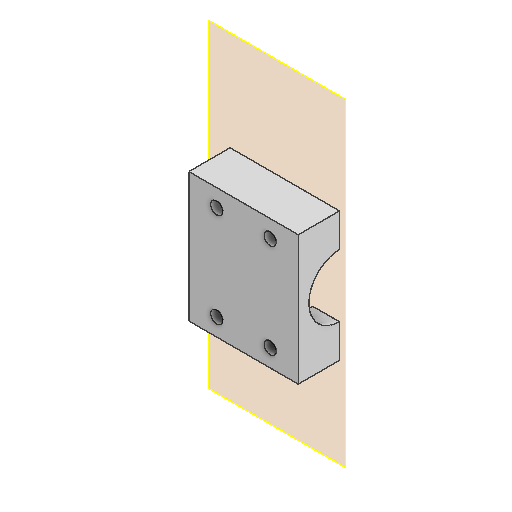
# Autodesk Inventor part: Cuvette Holder Transmit Holddown
Saved by Autodesk Inventor 2025.1 (Build 291241020, 241B)
## iProperties
Created: 2024-09-23
Part Number: Cuvette Holder Transmit Holddown
Material: Generic
Document SubType Name: Modeling
Designer: wayneslade
Density: 1 g/cm^3
Appearance: Default
Author: wayneslade
Autodesk Inventor part; units mm, degrees
ref_plane "YZ Plane" through (0, 0, 0) normal (1, 0, 0) x (0, 1, 0)
ref_plane "XZ Plane" through (0, 0, 0) normal (0, 1, 0) x (-1, 0, 0)
ref_plane "Work Plane1" through (0, 0, 0) normal (0, 0, 1) x (1, 0, 0)
sketch "Sketch1" plane through (0, 0, 0) normal (0, 0, 1) x (1, 0, 0)
  circle A0 centre (13.9438, -25.4) radius 3.3782 construction
  line L0 (31.1796, -40) -> (-0.106, -40) construction
  line L1 (31.1796, -40) -> (31.1796, -8.95) construction
  line L2 (31.1796, -8.95) -> (23.5548, -8.95) construction
  line L3 (23.5548, -8.95) -> (23.5548, -10.525) construction
  line L4 (23.5548, -10.525) -> (12.648, -10.525) construction
  line L5 (12.648, -10.525) -> (12.648, -8.95) construction
  line L6 (12.648, -8.95) -> (-0.106, -8.95) construction
  line L7 (-0.106, -8.95) -> (-0.106, -40) construction
  circle A1 centre (13.9438, 25.4) radius 3.3782 construction
  line L8 (-0.106, 8.95) -> (12.648, 8.95) construction
  line L9 (12.648, 8.95) -> (12.648, 10.525) construction
  line L10 (12.648, 10.525) -> (23.5548, 10.525) construction
  line L11 (23.5548, 10.525) -> (23.5548, 8.95) construction
  line L12 (23.5548, 8.95) -> (31.1796, 8.95) construction
  line L13 (31.1796, 8.95) -> (31.1796, 45) construction
  line L14 (-0.106, 45) -> (31.1796, 45) construction
  line L15 (-0.106, 45) -> (-0.106, 8.95) construction
  line L16 (31.1796, -18.5) -> (-0.106, -18.5)
  line L17 (-0.106, -18.5) -> (-0.106, 18.5)
  line L18 (-0.106, 18.5) -> (31.1796, 18.5)
  line L19 (31.1796, 18.5) -> (31.1796, -18.5)
  line L20 (65.998, 0) -> (-177.7308, 0) construction
  circle A2 centre (13.9438, 25.4) radius 5.5 construction
  circle A3 centre (23.1796, -13.5) radius 2 projected
  circle A4 centre (7.894, -13.5) radius 2 projected
  circle A5 centre (7.894, 13.5) radius 2 projected
  circle A6 centre (23.1796, 13.5) radius 2 projected
  point P0 (0, 0)
  point P1 (13.9438, 22.0218)
  dimension "d2" = 37
  dimension "d3" = 11
  constraints: 10 end point, 2 collinear, 2 horizontal, 2 parallel, 1 centre point, 1 coincident, 1 perpendicular, 1 vertical alignment, 4 other
  measures "d2" distance of L18.end L16.start
  measures "d3" diameter of A2
ref_plane "Work Plane2" through (-142.9124, -40, 12) normal (0, 0, 1) x (1, 0, 0)
extrude "Extrusion1" add sketch "Sketch1" along normal up to surface (12 mm away) contours L16 L17 L18 L19 | A3 | A4 | A5 | A6
sketch "Sketch2" plane through (0, 0, 0) normal (0, 1, 0) x (-1, 0, 0)
  line L0 (1.106, -8.95) -> (1.106, 0)
  line L1 (1.106, 0) -> (-32.1796, 0)
  line L2 (-32.1796, 0) -> (-32.1796, -8.95)
  line L3 (-38.8367, 0) -> (7.7631, 0) construction
  line L4 (-31.1796, -8.95) -> (-31.1796, 0) construction
  line L5 (0.106, 7.5245) -> (0.106, -7.5245) construction
  line L6 (-31.1796, -8.95) -> (-23.5548, -8.95)
  line L7 (-23.5548, -10.525) -> (-12.648, -10.525)
  line L8 (-12.648, -8.95) -> (0.106, -8.95)
  line L9 (-31.1796, -8.95) -> (-32.1796, -8.95)
  line L10 (0.106, -8.95) -> (1.106, -8.95)
  line L11 (-23.5548, -8.95) -> (-23.5548, -10.525)
  line L12 (-12.648, -8.95) -> (-12.648, -10.525)
  point P0 (0, 0)
  point P1 (1.106, 0)
  point P2 (-32.1796, 0)
  dimension "d7" = 1
  dimension "d8" = 1
  constraints: 20 end point, 4 collinear, 3 horizontal, 1 parallel, 1 perpendicular, 6 other
  measures "d7" distance between parallel lines of L4 L2
  measures "d8" distance between parallel lines of L0 L5
revolve "Revolution1" cut sketch "Sketch2" angle 360 about axis through (0, 0, 0) along (-1, 0, 0)
sketch "Sketch3" plane through (0, 0, 0) normal (0, 0, -1) x (-1, 0, 0)
  line L0 (0.106, 18.5) -> (-31.1796, 18.5)
  line L1 (-31.1796, 18.5) -> (-31.1796, -18.5)
  line L2 (-31.1796, -18.5) -> (0.106, -18.5)
  line L3 (0.106, -18.5) -> (0.106, 18.5)
  point P0 (0, 0)
  constraints: 8 end point, 2 coincident, 2 parallel, 1 horizontal, 1 perpendicular
extrude "Extrusion2" cut sketch "Sketch3" against normal blind 0.2
sketch "Sketch4" plane through (-0.106, 18.5, 12) normal (0, 0, 1) x (1, 0, 0)
  line L0 (31.2856, 0) -> (31.2856, -37) construction
  line L1 (0, 0) -> (31.2856, 0) construction
  line L2 (0, -37) -> (0, 0) construction
  line L3 (31.2856, -37) -> (0, -37) construction
  line L4 (31.2856, -5) -> (0, -5) construction
  line L5 (-6.2571, -18.5) -> (37.5427, -18.5) construction
  line L6 (31.2856, 0) -> (31.2856, -37) construction
  line L7 (0, -37) -> (0, 0) construction
  point P0 (0.106, -18.5)
  point P1 (23.2856, -5)
  point P2 (8, -5)
  point P3 (23.2856, -32)
  point P4 (8, -32)
  dimension "d12" = 8
  dimension "d13" = 8
  dimension "d14" = 5
  constraints: 4 point on line, 2 end point, 2 symmetric about line, 1 parallel
  measures "d12" distance from line of L0 point (23.286, -5)
  measures "d13" distance from line of L2 point (8, -5)
  measures "d14" distance between parallel lines of L1 L4
hole "Thru Hole Holddown Screws M3" at (23.1796, 13.5, 12) at (7.894, 13.5, 12) at (23.1796, -13.5, 12) at (7.894, -13.5, 12) direction (0, 0, -1) diameter 3.5 end through all
equation "\"d13\" = d12"
body "Solid1"
